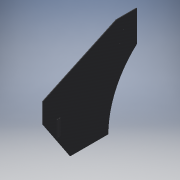
# Autodesk Inventor part: end_plate
Saved by Autodesk Inventor 2018.1 (Build 221171000, 171)
## iProperties
Created: 2017-10-22
Part Number: end_plate
Material: CFRP
Document SubType Name: Modeling
Designer: ku_sk
Density: 1.43 g/cm^3
Appearance: カーボンファイバー
Mass: 2260.49 g
Surface Area: 6541.63 cm^2
Volume: 1580.77 cm^3
Author: ku_sk
Autodesk Inventor part; units mm, degrees
ref_plane "YZ Plane" through (0, 0, 0) normal (1, 0, 0) x (0, 1, 0)
ref_plane "XY Plane" through (0, 0, 0) normal (0, 0, 1) x (1, 0, 0)
sketch "スケッチ1" plane through (0, 0, 0) normal (1, 0, 0) x (0, 1, 0)
  line L0 (-700, 210) -> (-700, 490)
  line L1 (-700, 490) -> (-400, 690)
  line L2 (-400, 690) -> (-250, 690)
  line L3 (-250, 690) -> (0, 150)
  line L4 (0, 150) -> (0, 0)
  line L5 (0, 0) -> (-230, 0)
  arc A0 (-230, 0) -> (-700, 210) centre (-700, -420.9524) ccw
  dimension "d0" = 690
  dimension "d1" = 280
  dimension "d2" = 200
  dimension "d3" = 300
  dimension "d4" = 150
  dimension "d5" = 700
  dimension "d6" = 230
  dimension "d7" = 150
  constraints: 12 end point, 2 perpendicular, 2 point on circle, 1 centre point, 1 coincident, 1 horizontal, 1 line through centre, 1 parallel
  measures "d0" distance between parallel lines of L5 L2
  measures "d1" distance of L0.start L0.end
  measures "d2" distance from line of L0.end L2
  measures "d3" distance from line of L1.end L0
  measures "d4" distance of L3.end L4.end
  measures "d5" distance between parallel lines of L0 L4
  measures "d6" distance of L4.end L5.end
  measures "d7" distance of L1.end L2.end
extrude "押し出し1" add sketch "スケッチ1" along normal blind 5
sketch "スケッチ2" plane through (5, 0, 0) normal (1, 0, 0) x (0, 0, -1)
  circle A0 centre (-100, -87) radius 2.5
  line L0 (0, 0) -> (-150, 0) projected
  line L1 (0, -230) -> (0, 0) projected
  circle A1 centre (-125, -164) radius 2.5
  dimension "d10" = 87
  dimension "d11" = 100
  dimension "d12" = 5
  dimension "d13" = 164
  dimension "d14" = 125
  dimension "d15" = 5
  constraints: 2 centre point
  measures "d10" distance from line of L0 A0.centre
  measures "d11" distance from line of L1 A0.centre
  measures "d12" diameter of A0
  measures "d13" distance from line of L0 A1.centre
  measures "d14" distance from line of L1 A1.centre
  measures "d15" diameter of A1
extrude "押し出し2" cut sketch "スケッチ2" against normal through all
ref_plane "作業平面1" through (0, -415, 0) normal (0, 1, 0) x (-1, 0, 0)
sketch "スケッチ6" plane through (0, -415, 0) normal (0, 1, 0) x (-1, 0, 0)
  line L0 (-10, 590) -> (-5, 575)
  line L1 (-10, 575) -> (-5, 560)
  line L2 (-5, 150) -> (-5, 690) projected
  line L3 (-10, 575) -> (-5.5, 576.5)
  line L4 (-10, 590) -> (-5, 591.6667)
  point P0 (0, 0)
  dimension "d48" = 15
  dimension "d55" = 15
  dimension "d56" = 15
  constraints: 8 end point, 3 point on line, 2 parallel, 1 perpendicular
  measures "d48" distance of L1.end L0.end
  measures "d55" vertical distance of L1.end L1.start
  measures "d56" vertical distance of L0.start L0.end
extrude "押し出し6" add sketch "スケッチ6" against normal blind 120
sketch "スケッチ7" plane through (5, -535, 591.6667) normal (0.3162, 0, 0.9487) x (0.9487, 0, -0.3162)
  line L0 (0, 0) -> (0, 120) projected
  line L1 (0, 118) -> (3.2705, 118)
  line L2 (3.2705, 118) -> (3.2705, 2)
  line L3 (3.2705, 2) -> (0, 2)
  line L4 (0, 2) -> (0, 118)
  line L5 (5.2705, 120) -> (5.2705, 0) projected
  line L6 (5.2705, 118) -> (8.0139, 118)
  line L7 (8.0139, 118) -> (8.0139, 2)
  line L8 (8.0139, 2) -> (5.2705, 2)
  line L9 (5.2705, 2) -> (5.2705, 118)
  line L10 (5.2705, 0) -> (0, 0) projected
  line L11 (10.0139, 120) -> (10.0139, 0) projected
  line L12 (0, 120) -> (5.2705, 120) projected
  point P0 (182.358, 535)
  dimension "d57" = 2
  dimension "d58" = 2
  dimension "d59" = 2
  dimension "d60" = 2
  constraints: 16 end point, 4 parallel, 3 point on line, 2 horizontal, 2 perpendicular, 1 collinear
  measures "d57" distance between parallel lines of L10 L3
  measures "d58" distance between parallel lines of L5 L2
  measures "d59" distance between parallel lines of L11 L7
  measures "d60" distance between parallel lines of L12 L1
extrude "押し出し7" cut sketch "スケッチ7" against normal through all contours L0 L1 L2 L3 | L5 L6 L7 L8
equation "\"d59\" = d58"
